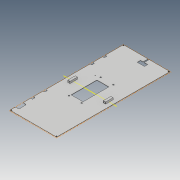
# Autodesk Inventor part: Screen Plate
Saved by Autodesk Inventor 2019 (Build 230136000, 136)
## iProperties
Created: 2020-09-21
Part Number: Screen Plate
Material: Generic
Document SubType Name: Modeling
Designer: giacomo
Density: 1 g/cm^3
Appearance: Default
Author: giacomo
Autodesk Inventor part; units mm, degrees
ref_plane "YZ Plane" through (0, 0, 0) normal (1, 0, 0) x (0, 1, 0)
ref_plane "XZ Plane" through (0, 0, 0) normal (0, 1, 0) x (-1, 0, 0)
ref_plane "XY Plane" through (0, 0, 0) normal (0, 0, 1) x (1, 0, 0)
sketch "Sketch1" plane through (0, 0, 0) normal (0, 1, 0) x (-1, 0, 0)
  line L0 (-90.1493, 193.0734) -> (34.8507, 193.0734) construction
  line L1 (34.8507, 193.0734) -> (34.8507, 51.5734) construction
  line L2 (34.8507, 51.5734) -> (28.8507, 51.5734) construction
  line L3 (28.8507, 51.5734) -> (28.8507, 31.5734) construction
  line L4 (34.8507, 31.5734) -> (28.8507, 31.5734) construction
  line L5 (34.8507, 31.5734) -> (34.8507, -109.9266) construction
  line L6 (34.8507, -109.9266) -> (-90.1493, -109.9266) construction
  line L7 (-90.1493, -109.9266) -> (-90.1493, 31.5734) construction
  line L8 (-90.1493, 31.5734) -> (-84.1493, 31.5734) construction
  line L9 (-84.1493, 51.5734) -> (-84.1493, 31.5734) construction
  line L10 (-90.1493, 51.5734) -> (-84.1493, 51.5734) construction
  line L11 (-90.1493, 51.5734) -> (-90.1493, 193.0734) construction
  line L12 (-91.6493, 194.5734) -> (-91.6493, -111.4266) construction
  line L13 (-91.6493, -111.4266) -> (36.3507, -111.4266) construction
  line L14 (36.3507, -111.4266) -> (36.3507, 194.5734) construction
  line L15 (36.3507, 194.5734) -> (-91.6493, 194.5734) construction
  circle A0 centre (-88.1493, -107.9266) radius 1.1 construction
  line L16 (-86.1493, -109.9266) -> (-90.1493, -109.9266) construction
  line L17 (-86.1493, -109.9266) -> (-86.1493, -105.9266) construction
  line L18 (-86.1493, -105.9266) -> (-90.1493, -105.9266) construction
  line L19 (-90.1493, -109.9266) -> (-90.1493, -105.9266) construction
  line L20 (34.8507, -109.9266) -> (30.8507, -109.9266) construction
  line L21 (34.8507, -105.9687) -> (34.8507, -109.9266) construction
  line L22 (34.8507, -105.9687) -> (30.8507, -105.9687) construction
  line L23 (30.8507, -105.9687) -> (30.8507, -109.9266) construction
  circle A1 centre (32.8507, -107.9687) radius 1.1 construction
  circle A2 centre (-88.1493, 191.0734) radius 1.1 construction
  line L24 (-90.1493, 189.0734) -> (-90.1493, 193.0734) construction
  line L25 (-90.1493, 189.0734) -> (-86.1493, 189.0734) construction
  line L26 (-86.1493, 189.0734) -> (-86.1493, 193.0734) construction
  line L27 (-90.1493, 193.0734) -> (-86.1493, 193.0734) construction
  circle A3 centre (32.8507, 191.0734) radius 1.1 construction
  line L28 (30.8507, 193.0734) -> (34.8507, 193.0734) construction
  line L29 (30.8507, 193.0734) -> (30.8507, 189.0734) construction
  line L30 (30.8507, 189.0734) -> (34.8507, 189.0734) construction
  line L31 (34.8507, 193.0734) -> (34.8507, 189.0734) construction
  point P0 (0, 0)
  point P1 (0, 0)
  constraints: 64 end point, 4 centre point
sketch "Sketch2" plane through (0, 0, 0) normal (0, 1, 0) x (-1, 0, 0)
  line L0 (-89.7618, 28.8226) -> (-89.7618, 191.8096)
  line L1 (-88.7618, 192.8096) -> (33.3754, 192.8096)
  line L2 (34.3754, 191.8096) -> (34.3754, -108.6932)
  line L3 (-89.7618, -108.6932) -> (-89.7618, 28.8226)
  circle A0 centre (-87.7618, -107.6932) radius 1
  circle A1 centre (32.3754, -107.6932) radius 1
  line L4 (34.3754, 28.9308) -> (34.3754, -108.6932)
  circle A2 centre (-87.7618, 190.8096) radius 1
  circle A3 centre (32.3754, 190.8096) radius 1
  arc A4 (34.3754, 191.8096) -> (33.3754, 192.8096) centre (33.3754, 191.8096) ccw
  arc A5 (-88.7618, 192.8096) -> (-89.7618, 191.8096) centre (-88.7618, 191.8096) ccw
  arc A6 (-89.7618, -108.6932) -> (-88.7618, -109.6932) centre (-88.7618, -108.6932) ccw
  arc A7 (33.3754, -109.6932) -> (34.3754, -108.6932) centre (33.3754, -108.6932) ccw
  line L5 (-43.6932, 76.0582) -> (-11.6932, 76.0582)
  line L6 (-11.6932, 76.0582) -> (-11.6932, 7.0582)
  line L7 (-11.6932, 7.0582) -> (-43.6932, 7.0582)
  line L8 (-43.6932, 7.0582) -> (-43.6932, 76.0582)
  circle A8 centre (-44.6932, 80.8582) radius 1.75
  circle A9 centre (-10.6932, 80.8582) radius 1.75
  circle A10 centre (-10.6932, -3.9418) radius 1.75
  circle A11 centre (-44.6932, -3.9418) radius 1.75
  line L9 (-43.8518, -87.5066) -> (-24.58, -87.5066)
  line L10 (-24.58, -87.5066) -> (-24.58, -96.4362)
  line L11 (-43.8518, -96.4362) -> (-43.8518, -87.5066)
  line L12 (-34.6195, -96.4362) -> (-34.6195, -109.6932)
  line L13 (-31.2888, -109.6932) -> (-31.2888, -96.4362)
  line L14 (-24.58, -96.4362) -> (-31.2888, -96.4362)
  line L15 (-34.6195, -96.4362) -> (-43.8518, -96.4362)
  line L16 (33.3754, -109.6932) -> (-31.2888, -109.6932)
  line L17 (-34.6195, -109.6932) -> (-88.7618, -109.6932)
  line L18 (34.0825, -109.4003) -> (-89.4689, 192.5167) construction
  line L19 (-89.4689, -109.4003) -> (34.0825, 192.5167) construction
  line L20 (-27.6932, 41.5582) -> (9.3943, 41.5582) construction
  point P0 (0, 0)
  point P1 (-89.7618, 188.8096)
  point P2 (-85.7618, 192.8096)
  point P3 (-89.7618, 192.8096)
  dimension "d3" = 1
  dimension "d47" = 69
  dimension "d48" = 32
  dimension "d52" = 34.5
  dimension "d53" = 16
  dimension "d54" = 3.5
  dimension "d55" = 3.5
  dimension "d56" = 3.5
  dimension "d57" = 3.5
  dimension "d59" = 0
  dimension "d62" = 0
  dimension "d64" = 0
  dimension "d65" = 0
  dimension "d66" = 11
  dimension "d67" = 4.8
  dimension "d68" = 1
  dimension "d69" = 1
  dimension "d87" = 2
  dimension "d88" = 2
  dimension "d89" = 2
  dimension "d90" = 2
  dimension "d91" = 2
  dimension "d92" = 2
  dimension "d93" = 2
  dimension "d94" = 2
  dimension "d95" = 2
  dimension "d96" = 2
  dimension "d97" = 2
  dimension "d98" = 2
  constraints: 42 end point, 12 centre point, 12 point on circle, 6 parallel, 3 equal radius, 3 horizontal, 3 point on line, 2 perpendicular, 2 tangent, 1 midpoint
  measures "d3" radius of A4
  measures "d47" distance of L7.end L5.start
  measures "d48" distance of L5.start L5.end
  measures "d52" distance between parallel lines of L7 L20
  measures "d53" distance from line of L8 L20.start
  measures "d54" diameter of A10
  measures "d55" diameter of A11
  measures "d56" diameter of A9
  measures "d57" diameter of A8
  measures "d59" horizontal distance of A9.centre A10.centre
  measures "d62" horizontal distance of A8.centre A11.centre
  measures "d64" vertical distance of A10.centre A11.centre
  measures "d65" vertical distance of A8.centre A9.centre
  measures "d66" distance from line of L7 A10.centre
  measures "d67" distance from line of L5 A9.centre
  measures "d68" distance from line of L6 A10.centre
  measures "d69" distance from line of L8 A11.centre
  measures "d87" distance from line of L1 A2.centre
  measures "d88" distance from line of L0 A2.centre
  measures "d89" diameter of A2
  measures "d90" distance from line of L1 A3.centre
  measures "d91" distance from line of L2 A3.centre
  measures "d92" diameter of A3
  measures "d93" distance from line of A0.centre L3
  measures "d94" distance from line of L17 A0.centre
  measures "d95" diameter of A0
  measures "d96" distance from line of L16 A1.centre
  measures "d97" distance from line of A1.centre L2
  measures "d98" diameter of A1
extrude "Extrusion1" add sketch "Sketch2" along normal blind 1
ref_plane "Work Plane1" through (-33.3754, 0, 41.5582) normal (0, 0, 1) x (1, 0, 0)
sketch "Sketch4" plane through (0, 1, 0) normal (0, 1, 0) x (1, 0, 0)
  line L0 (79.1186, -31.5582) -> (73.1186, -31.5582)
  line L1 (73.1186, -31.5582) -> (73.1186, -51.5582)
  line L2 (73.1186, -51.5582) -> (79.1186, -51.5582)
  line L3 (79.1186, -51.5582) -> (79.1186, -31.5582)
  line L4 (117.2493, -41.5582) -> (-61.9507, -41.5582) projected
  line L5 (-15.9231, -31.5582) -> (-21.9231, -31.5582)
  line L6 (-21.9231, -31.5582) -> (-21.9231, -51.5582)
  line L7 (-21.9231, -51.5582) -> (-15.9231, -51.5582)
  line L8 (-15.9231, -51.5582) -> (-15.9231, -31.5582)
  dimension "d10" = 6
  dimension "d11" = 20
  dimension "d12" = 10
  dimension "d13" = 6
  dimension "d14" = 20
  dimension "d15" = 10
  constraints: 16 end point, 4 parallel, 2 horizontal, 2 perpendicular
  measures "d10" distance of L2.end L1.end
  measures "d11" distance of L1.end L0.end
  measures "d12" distance between parallel lines of L4 L0
  measures "d13" distance of L6.end L7.end
  measures "d14" distance of L7.end L5.start
  measures "d15" distance between parallel lines of L5 L4
extrude "Extrusion2" add sketch "Sketch4" along normal blind 5
sketch "Sketch6" plane through (-21.9231, 1, 51.5582) normal (0, 0, 1) x (1, 0, 0)
  line L0 (0, 5) -> (6, 5) projected
  line L1 (0, 0) -> (0, 5) projected
  line L2 (95.0417, 5) -> (101.0417, 5) projected
  line L3 (95.0417, 0) -> (95.0417, 5) projected
  point P0 (21.9231, -1)
  point P1 (3, 2.5)
  point P2 (98.0417, 2.5)
  dimension "d22" = 2.5
  dimension "d23" = 3
  dimension "d24" = 2.5
  dimension "d25" = 3
  measures "d22" distance from line of L0 point (3, 2.5)
  measures "d23" distance from line of L1 point (3, 2.5)
  measures "d24" distance from line of L2 point (98.042, 2.5)
  measures "d25" distance from line of L3 point (98.042, 2.5)
hole "Hole1" at (-18.9231, 3.5, 51.5582) at (76.1186, 3.5, 51.5582) direction (0, 0, -1) diameter 2.6 depth 5 countersink diameter 5 countersink angle 82
sketch "Sketch7" plane through (-18.9231, 3.5, 46.5582) normal (0, 0, 1) x (1, 0, 0)
  circle A0 centre (0, 0) radius 1.3 projected
  point P0 (18.9231, -3.5)
  constraints: 1 coincident
hole "Hole2" at (-18.9231, 3.5, 46.5582) direction (0, 0, -1) diameter 2.6 depth 15 tip angle 118
sketch "Sketch8" plane through (76.1186, 3.5, 46.5582) normal (0, 0, 1) x (1, 0, 0)
  circle A0 centre (0, 0) radius 1.3 projected
  point P0 (-76.1186, -3.5)
  constraints: 1 coincident
hole "Hole3" at (76.1186, 3.5, 46.5582) direction (0, 0, -1) diameter 2.6 depth 15 tip angle 118
sketch "Sketch9" plane through (0, 0, 0) normal (0, -1, 0) x (1, 0, 0)
  line L0 (-34.3754, -108.6932) -> (-34.3754, 191.8096) projected
  line L1 (-34.3754, 137.8096) -> (-30.8754, 137.8096)
  line L2 (-29.8754, 136.8096) -> (-29.8754, 131.8096)
  line L3 (-30.8754, 130.8096) -> (-34.3754, 130.8096)
  line L4 (-34.3754, 130.8096) -> (-34.3754, 137.8096)
  line L5 (-34.3754, 104.8096) -> (-30.8754, 104.8096)
  line L6 (-29.8754, 103.8096) -> (-29.8754, 98.8096)
  line L7 (-30.8754, 97.8096) -> (-34.3754, 97.8096)
  line L8 (-34.3754, 97.8096) -> (-34.3754, 104.8096)
  line L9 (-34.3754, -21.1904) -> (-30.8754, -21.1904)
  line L10 (-29.8754, -22.1904) -> (-29.8754, -27.1904)
  line L11 (-30.8754, -28.1904) -> (-34.3754, -28.1904)
  line L12 (-34.3754, -28.1904) -> (-34.3754, -21.1904)
  line L13 (-34.3754, -54.1904) -> (-30.8754, -54.1904)
  line L14 (-29.8754, -55.1904) -> (-29.8754, -60.1904)
  line L15 (-30.8754, -61.1904) -> (-34.3754, -61.1904)
  line L16 (-34.3754, -61.1904) -> (-34.3754, -54.1904)
  line L17 (-33.3754, 192.8096) -> (88.7618, 192.8096) projected
  arc A0 (-29.8754, 136.8096) -> (-30.8754, 137.8096) centre (-30.8754, 136.8096) ccw
  arc A1 (-30.8754, 130.8096) -> (-29.8754, 131.8096) centre (-30.8754, 131.8096) ccw
  arc A2 (-29.8754, 103.8096) -> (-30.8754, 104.8096) centre (-30.8754, 103.8096) ccw
  arc A3 (-30.8754, 97.8096) -> (-29.8754, 98.8096) centre (-30.8754, 98.8096) ccw
  arc A4 (-29.8754, -22.1904) -> (-30.8754, -21.1904) centre (-30.8754, -22.1904) ccw
  arc A5 (-30.8754, -28.1904) -> (-29.8754, -27.1904) centre (-30.8754, -27.1904) ccw
  arc A6 (-29.8754, -55.1904) -> (-30.8754, -54.1904) centre (-30.8754, -55.1904) ccw
  arc A7 (-30.8754, -61.1904) -> (-29.8754, -60.1904) centre (-30.8754, -60.1904) ccw
  point P0 (0, 0)
  point P1 (-29.8754, 97.8096)
  point P2 (-29.8754, 104.8096)
  point P3 (-29.8754, -28.1904)
  point P4 (-29.8754, -21.1904)
  point P5 (-29.8754, -61.1904)
  point P6 (-29.8754, -54.1904)
  dimension "d70" = 55
  dimension "d71" = 7
  dimension "d72" = 7
  dimension "d73" = 26
  dimension "d74" = 26
  dimension "d75" = 7
  dimension "d76" = 7
  dimension "d77" = 119
  dimension "d78" = 4.5
  dimension "d79" = 4.5
  dimension "d80" = 1
  dimension "d81" = 1
  constraints: 32 end point, 18 point on line, 16 point on circle, 16 tangent, 8 centre point, 8 parallel, 6 equal radius, 4 horizontal, 4 perpendicular
  measures "d70" distance between parallel lines of L1 L17
  measures "d71" distance between parallel lines of L3 L1
  measures "d72" distance of point (-29.875, 104.81) point (-29.875, 97.81)
  measures "d73" distance between parallel lines of L5 L3
  measures "d74" distance between parallel lines of L13 L11
  measures "d75" distance of point (-29.875, -21.19) point (-29.875, -28.19)
  measures "d76" distance of point (-29.875, -54.19) point (-29.875, -61.19)
  measures "d77" distance between parallel lines of L9 L7
  measures "d78" distance between parallel lines of L0 L2
  measures "d79" distance of L9.start point (-29.875, -21.19)
  measures "d80" radius of A0
  measures "d81" radius of A1
extrude "Extrusion3" cut sketch "Sketch9" against normal through all
fillet "Fillet1" radius 2 8 edges at (-34.3754, 0.5, 137.8096) (-34.3754, 0.5, 130.8096) (-34.3754, 0.5, 104.8096) (-34.3754, 0.5, 97.8096) (-34.3754, 0.5, -21.1904) (-34.3754, 0.5, -28.1904) (-34.3754, 0.5, -54.1904) (-34.3754, 0.5, -61.1904)
sketch "Sketch10" plane through (-33.3754, 0, 41.5582) normal (0, 0, 1) x (1, 0, 0)
  line L0 (158.018, -104.466) -> (-19.6119, -104.466)
  line L1 (-19.6119, -104.466) -> (-19.6119, 75.8038)
  line L2 (-19.6119, 75.8038) -> (158.018, 75.8038)
  line L3 (158.018, 75.8038) -> (158.018, -104.466)
  point P0 (33.3754, 0)
  constraints: 8 end point, 2 parallel, 1 horizontal, 1 perpendicular
extrude "Extrusion4" [suppressed]
sketch "Sketch11" plane through (0, 0, 0) normal (0, -1, 0) x (1, 0, 0)
  line L0 (-34.3754, 139.8096) -> (-34.3754, 191.8096) projected
  line L1 (-34.3754, 178.177) -> (-25.2482, 178.177)
  line L2 (-25.2482, 178.177) -> (-25.2482, 158.3724)
  line L3 (-25.2482, 158.3724) -> (-34.3754, 158.3724)
  line L4 (-34.3754, 158.3724) -> (-34.3754, 178.177)
  point P0 (0, 0)
  constraints: 8 end point, 2 parallel, 1 horizontal, 1 perpendicular, 1 point on line
extrude "Extrusion5" cut sketch "Sketch11" against normal through all
fillet "Fillet2" radius 3 4 edges at (-34.3754, 0.5, 178.177) (-25.2482, 0.5, 178.177) (-25.2482, 0.5, 158.3724) (-34.3754, 0.5, 158.3724)
body "Solid1"
